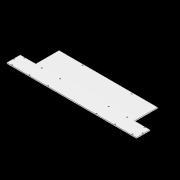
# Autodesk Inventor part: TopBottomUHMW
Saved by Autodesk Inventor 2021 (Build 250183000, 183)
## iProperties
Created: 2021-03-10
Part Number: TopBottomUHMW
Material: UHMW, White
Document SubType Name: Modeling
Designer: Dylan
Density: 0.94 g/cm^3
Appearance: Smooth - White
Mass: 3188.13 g
Surface Area: 7467.87 cm^2
Volume: 3391.63 cm^3
Author: Dylan
Autodesk Inventor part; units mm, degrees
ref_plane "YZ Plane" through (0, 0, 0) normal (1, 0, 0) x (0, 1, 0)
ref_plane "XZ Plane" through (0, 0, 0) normal (0, 1, 0) x (-1, 0, 0)
sketch "Sketch1" plane through (0, 0, 0) normal (0, 1, 0) x (-1, 0, 0)
  line L0 (0, 0) -> (1219.2, 0)
  line L1 (1219.2, 0) -> (1219.2, -345.44)
  line L2 (1219.2, -345.44) -> (0, -345.44)
  line L3 (0, -345.44) -> (0, 0)
  line L4 (1219.2, -345.44) -> (1073.15, -345.44)
  line L5 (1073.15, -345.44) -> (1073.15, -152.4)
  line L6 (1073.15, -152.4) -> (1219.2, -152.4)
  line L7 (1219.2, -152.4) -> (1219.2, -345.44)
  line L8 (0, -345.44) -> (146.05, -345.44)
  line L9 (146.05, -345.44) -> (146.05, -152.4)
  line L10 (146.05, -152.4) -> (0, -152.4)
  line L11 (0, -152.4) -> (0, -345.44)
  dimension "d0" = 1219.2
  dimension "d1" = 345.44
  dimension "d3" = 152.4
  dimension "d4" = 146.05
  constraints: 24 end point, 6 parallel, 3 horizontal, 3 perpendicular, 1 collinear, 1 point on line
  measures "d0" distance of L1.end L2.end
  measures "d1" distance of L0.end L1.end
  measures "d3" distance between parallel lines of L0 L6
  measures "d4" distance of L5.end L6.end
extrude "Extrusion1" add sketch "Sketch1" along normal blind 9.525 contours L0 L1 L6 L5 L2 L9 L10 L3
sketch "Sketch2" plane through (0, 0, 0) normal (0, -1, 0) x (1, 0, 0)
  line L0 (-51.1937, -114.3) -> (-51.1937, -127) projected
  line L1 (-37.7063, -127) -> (-51.1937, -127) projected
  line L2 (-37.7063, -114.3) -> (-37.7063, -127) projected
  line L3 (-51.1937, -114.3) -> (-37.7063, -114.3) projected
  line L4 (-214.7062, -114.3) -> (-214.7062, -127) projected
  line L5 (-201.2188, -127) -> (-214.7062, -127) projected
  line L6 (-201.2188, -114.3) -> (-201.2188, -127) projected
  line L7 (-214.7062, -114.3) -> (-201.2188, -114.3) projected
  line L8 (-384.5687, -320.04) -> (-384.5687, -345.44) projected
  line L9 (-371.0813, -345.44) -> (-384.5687, -345.44) projected
  line L10 (-371.0813, -320.04) -> (-371.0813, -345.44) projected
  line L11 (-384.5687, -320.04) -> (-371.0813, -320.04) projected
  line L12 (-848.1187, -320.04) -> (-848.1187, -345.44) projected
  line L13 (-834.6313, -345.44) -> (-848.1187, -345.44) projected
  line L14 (-834.6313, -320.04) -> (-834.6313, -345.44) projected
  line L15 (-848.1187, -320.04) -> (-834.6313, -320.04) projected
  line L16 (-1181.4937, -114.3) -> (-1181.4937, -127) projected
  line L17 (-1168.0063, -127) -> (-1181.4937, -127) projected
  line L18 (-1168.0063, -114.3) -> (-1168.0063, -127) projected
  line L19 (-1181.4937, -114.3) -> (-1168.0063, -114.3) projected
  line L20 (-1206.5, -56.7563) -> (-1219.2, -56.7563) projected
  line L21 (-1219.2, -70.2437) -> (-1219.2, -56.7563) projected
  line L22 (-1206.5, -70.2437) -> (-1219.2, -70.2437) projected
  line L23 (-1206.5, -56.7563) -> (-1206.5, -70.2437) projected
  line L24 (-1017.9812, -114.3) -> (-1017.9812, -127) projected
  line L25 (-1004.4938, -127) -> (-1017.9812, -127) projected
  line L26 (-1004.4938, -114.3) -> (-1004.4938, -127) projected
  line L27 (-1017.9812, -114.3) -> (-1004.4938, -114.3) projected
  line L28 (0, -56.7563) -> (-12.7, -56.7563) projected
  line L29 (-12.7, -70.2437) -> (-12.7, -56.7563) projected
  line L30 (0, -70.2437) -> (-12.7, -70.2437) projected
  line L31 (0, -56.7563) -> (0, -70.2437) projected
  line L32 (-375.8438, -12.7) -> (-375.8438, 0) projected
  line L33 (-389.3312, 0) -> (-375.8438, 0) projected
  line L34 (-389.3312, -12.7) -> (-389.3312, 0) projected
  line L35 (-375.8438, -12.7) -> (-389.3312, -12.7) projected
  line L36 (-949.325, 0) -> (-949.325, -12.7) projected
  line L37 (-962.025, -12.7) -> (-949.325, -12.7) projected
  line L38 (-962.025, 0) -> (-962.025, -12.7) projected
  line L39 (-949.325, 0) -> (-962.025, 0) projected
  line L40 (-1181.4937, -127) -> (-1168.0063, -114.3) construction
  line L41 (-1181.4937, -114.3) -> (-1168.0063, -127) construction
  line L42 (-1206.5, -70.2437) -> (-1219.2, -56.7563) construction
  line L43 (-1206.5, -56.7563) -> (-1219.2, -70.2437) construction
  line L44 (-962.025, -12.7) -> (-949.325, 0) construction
  line L45 (-949.325, -12.7) -> (-962.025, 0) construction
  line L46 (-848.1187, -320.04) -> (-834.6313, -345.44) construction
  line L47 (-848.1187, -345.44) -> (-834.6313, -320.04) construction
  line L48 (-375.8438, -12.7) -> (-389.3312, 0) construction
  line L49 (-389.3312, -12.7) -> (-375.8438, 0) construction
  line L50 (-214.7062, -127) -> (-201.2188, -114.3) construction
  line L51 (-214.7062, -114.3) -> (-201.2188, -127) construction
  line L52 (-51.1937, -127) -> (-37.7063, -114.3) construction
  line L53 (-51.1937, -114.3) -> (-37.7063, -127) construction
  line L54 (-12.7, -70.2437) -> (0, -56.7563) construction
  line L55 (-12.7, -56.7563) -> (0, -70.2437) construction
  line L56 (-384.5687, -345.44) -> (-371.0813, -320.04) construction
  line L57 (-384.5687, -320.04) -> (-371.0813, -345.44) construction
  line L58 (-1017.9812, -127) -> (-1004.4938, -114.3) construction
  line L59 (-1017.9812, -114.3) -> (-1004.4938, -127) construction
  circle A0 centre (-836.6125, -6.35) radius 5.0419
  circle A1 centre (-1011.2375, -6.35) radius 5.0419
  circle A2 centre (-1174.75, -6.35) radius 5.0419
  circle A3 centre (-1212.85, -63.5) radius 5.0419
  circle A4 centre (-1174.75, -120.65) radius 5.0419
  circle A5 centre (-1011.2375, -120.65) radius 5.0419
  circle A6 centre (-836.6125, -120.65) radius 5.0419
  circle A7 centre (-382.5875, -6.35) radius 5.0419
  line L60 (0, 0) -> (0, -152.4) projected
  line L61 (-1219.2, 0) -> (0, 0) projected
  line L62 (-1219.2, -152.4) -> (-1219.2, 0) projected
  line L63 (-1073.15, -152.4) -> (-1219.2, -152.4) projected
  line L64 (-1073.15, -345.44) -> (-1073.15, -152.4) projected
  line L65 (-146.05, -345.44) -> (-1073.15, -345.44) projected
  line L66 (-146.05, -152.4) -> (-146.05, -345.44) projected
  line L67 (0, -152.4) -> (-146.05, -152.4) projected
  circle A8 centre (-207.9625, -6.35) radius 5.0419
  circle A9 centre (-44.45, -6.35) radius 5.0419
  circle A10 centre (-44.45, -120.65) radius 5.0419
  circle A11 centre (-207.9625, -120.65) radius 5.0419
  line L68 (0, 0) -> (0, -152.4) projected
  line L69 (0, 0) -> (0, -152.4) projected
  circle A12 centre (-6.35, -63.5) radius 5.0419
  circle A13 centre (-382.5875, -120.65) radius 5.0419
  circle A14 centre (-841.375, -332.74) radius 5.0419
  circle A15 centre (-377.825, -332.74) radius 5.0419
  point P0 (-1212.85, -63.5)
  point P1 (-1174.75, -120.65)
  point P2 (-1011.2375, -120.65)
  point P3 (-955.675, -6.35)
  point P4 (-841.375, -332.74)
  point P5 (-377.825, -332.74)
  point P6 (-207.9625, -120.65)
  point P7 (-44.45, -120.65)
  point P8 (-6.35, -63.5)
  point P9 (-382.5875, -6.35)
  constraints: 40 end point, 16 centre point, 10 midpoint, 8 perpendicular, 6 parallel, 32 other
hole "Hole1" at (-1212.85, 0, -63.5) at (-1174.75, 0, -120.65) at (-1011.2375, 0, -120.65) at (-841.375, 0, -332.74) at (-377.825, 0, -332.74) at (-207.9625, 0, -120.65) at (-44.45, 0, -120.65) at (-6.35, 0, -63.5) at (-382.5875, 0, -6.35) at (-1011.2375, 0, -6.35) at (-1174.75, 0, -6.35) at (-836.6125, 0, -6.35) at (-836.6125, 0, -120.65) at (-382.5875, 0, -120.65) at (-207.9625, 0, -6.35) at (-44.45, 0, -6.35) direction (0, 1, 0) diameter 10.0838 end through all clearance for "Hex Head Bolt" size "3/8" standard "Ansi Unified Screw Threads"
ref_plane "Work Plane1" through (-1073.15, 68.2625, -229.87) normal (-1, 0, 0) x (0, 0, -1)
sketch "Sketch3" plane through (0, 0, 0) normal (0, -1, 0) x (1, 0, 0)
  line L0 (0, -152.4) -> (-146.05, -152.4) projected
  line L1 (-146.05, -127) -> (0, -127)
  line L2 (0, -127) -> (0, -152.4)
  line L3 (0, -152.4) -> (-146.05, -152.4)
  line L4 (-146.05, -152.4) -> (-146.05, -127)
  line L5 (-1073.15, -152.4) -> (-1219.2, -152.4) projected
  line L6 (-1219.2, -152.4) -> (-1073.15, -152.4)
  line L7 (-1073.15, -152.4) -> (-1073.15, -127)
  line L8 (-1073.15, -127) -> (-1219.2, -127)
  line L9 (-1219.2, -127) -> (-1219.2, -152.4)
  point P0 (0, 0)
  point P1 (-1206.5, -127)
  constraints: 16 end point, 4 parallel, 3 point on line, 2 perpendicular, 1 horizontal, 2 other
extrude "Extrusion2" cut sketch "Sketch3" against normal through all
body "Solid1"
